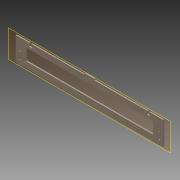
# Autodesk Inventor part: Panel_front
Saved by Autodesk Inventor 2013 (Build 170138000, 138)
## iProperties
Created: 2013-02-02
Part Number: Panel_front
Material: Aluminum 6061
Document SubType Name: Modeling
Designer: xylzlyx
Density: 1 g/cm^3
Author: xylzlyx
Autodesk Inventor part; units mm, degrees
ref_plane "YZ Plane" through (0, 0, 0) normal (1, 0, 0) x (0, 1, 0)
ref_plane "XZ Plane" through (0, 0, 0) normal (0, 1, 0) x (-1, 0, 0)
ref_plane "XY Plane" through (0, 0, 0) normal (0, 0, 1) x (1, 0, 0)
ref_plane "Work Plane1" through (0, 0, -9.525) normal (0, 0, 1) x (1, 0, 0)
sketch "Sketch1" plane through (0, 0, -9.525) normal (0, 0, 1) x (1, 0, 0)
  line L0 (381, -60.8043) -> (381, -64.0283) construction
  line L1 (381, -64.0283) -> (0, -64.0283) construction
  line L2 (0, -64.0283) -> (0, -60.8043) construction
  line L3 (0, -60.8043) -> (381, -60.8043) construction
  line L4 (381, 0) -> (0, 0) construction
  line L5 (0, 0) -> (0, 3.175) construction
  line L6 (0, 3.175) -> (381, 3.175) construction
  line L7 (381, 3.175) -> (381, 0) construction
  line L8 (381, -60.8043) -> (0, -60.8043)
  line L9 (0, -60.8043) -> (0, 0)
  line L10 (0, 0) -> (381, 0)
  line L11 (381, 0) -> (381, -60.8043)
  constraints: 24 end point, 5 horizontal, 4 coincident, 4 vertical, 2 parallel, 1 perpendicular, 8 other
extrude "FrontPanel" add sketch "Sketch1" against normal blind 3.175
fillet "CornerFillet" radius 1 4 edges at (381, -60.8043, -11.1125) (0, -60.8043, -11.1125) (0, 0, -11.1125) (381, 0, -11.1125)
sketch "ScrewSlotSketch" plane through (0, 0, -9.525) normal (0, 0, 1) x (1, 0, 0)
  line L0 (368.3, -28.0035) -> (368.3, -1) projected
  line L1 (12.7, -1) -> (12.7, -28.0035) projected
  line L2 (381, 0) -> (0, 0) construction
  line L3 (0, 0) -> (0, 3.175) construction
  line L4 (0, 3.175) -> (381, 3.175) construction
  line L5 (381, 3.175) -> (381, 0) construction
  line L6 (381, -60.8043) -> (381, -64.0283) construction
  line L7 (381, -64.0283) -> (0, -64.0283) construction
  line L8 (0, -64.0283) -> (0, -60.8043) construction
  line L9 (0, -60.8043) -> (381, -60.8043) construction
  line L10 (344.7987, -8.89) -> (344.7987, 3.175)
  line L11 (344.7987, 3.175) -> (341.0014, 3.175)
  line L12 (341.0014, 3.175) -> (341.0014, -8.89)
  line L13 (341.0014, -8.89) -> (344.7987, -8.89)
  line L14 (346.9958, -8.89) -> (338.8043, -8.89)
  line L15 (338.8043, -8.89) -> (338.8043, -5.8579)
  line L16 (338.8043, -5.8579) -> (346.9958, -5.8579)
  line L17 (346.9958, -5.8579) -> (346.9958, -8.89)
  line L18 (36.2014, -8.89) -> (39.9987, -8.89)
  line L19 (39.9987, -8.89) -> (39.9987, 3.175)
  line L20 (39.9987, 3.175) -> (36.2014, 3.175)
  line L21 (36.2014, 3.175) -> (36.2014, -8.89)
  line L22 (34.0043, -8.89) -> (42.1958, -8.89)
  line L23 (42.1958, -8.89) -> (42.1958, -5.8579)
  line L24 (42.1958, -5.8579) -> (34.0043, -5.8579)
  line L25 (34.0043, -5.8579) -> (34.0043, -8.89)
  point P0 (342.9, 3.175)
  point P1 (342.9, -8.89)
  point P2 (38.1, -8.89)
  point P3 (38.1, 3.175)
  dimension "d4" = 12.065
  dimension "d6" = 3.7973
  dimension "d7" = 25.4
  dimension "d8" = 8.1915
  dimension "d9" = 3.0321
  dimension "d10" = 3.7973
  dimension "d11" = 12.065
  dimension "d12" = 8.1915
  dimension "d13" = 3.0321
  dimension "d14" = 25.4
  constraints: 48 end point, 11 parallel, 6 horizontal, 6 midpoint, 4 vertical, 2 perpendicular, 2 point on line, 1 collinear, 7 other
  measures "d4" distance of L10.start L10.end
  measures "d6" distance of L10.end L11.end
  measures "d7" distance from line of L0 point (342.9, 3.175)
  measures "d8" distance of L14.start L14.end
  measures "d9" distance of L14.end L15.end
  measures "d10" distance of L19.end L20.end
  measures "d11" distance of L20.end L18.start
  measures "d12" distance of L22.start L22.end
  measures "d13" distance of L22.end L23.end
  measures "d14" distance from line of L1 point (38.1, 3.175)
extrude "ScrewSlotExtrusion" cut sketch "ScrewSlotSketch" against normal blind 3.175
fillet "ScrewSlotFillet" radius 0.5 16 edges at (344.7987, 0, -11.1125) (341.0014, 0, -11.1125) (344.7987, -5.8579, -11.1125) (341.0014, -5.8579, -11.1125) (338.8043, -5.8579, -11.1125) (338.8043, -8.89, -11.1125) (346.9958, -8.89, -11.1125) (346.9958, -5.8579, -11.1125) (42.1958, -8.89, -11.1125) (42.1958, -5.8579, -11.1125) (39.9987, -5.8579, -11.1125) (39.9987, 0, -11.1125) (36.2014, 0, -11.1125) (36.2014, -5.8579, -11.1125) (34.0043, -5.8579, -11.1125) (34.0043, -8.89, -11.1125)
sketch "ScrewHoleSketch" plane through (0, 0, -9.525) normal (0, 0, 1) x (1, 0, 0)
  line L0 (34.0043, -8.39) -> (34.0043, -6.3579) projected
  line L1 (368.3, -28.5035) -> (371.475, -28.5035) projected
  line L2 (371.475, -32.3008) -> (368.3, -32.3008) projected
  line L3 (9.525, -28.5035) -> (12.7, -28.5035) projected
  line L4 (12.7, -32.3008) -> (9.525, -32.3008) projected
  line L5 (371.475, -28.5035) -> (371.475, -32.3008) construction
  line L6 (9.525, -28.5035) -> (9.525, -32.3008) construction
  point P0 (0, 0)
  point P1 (11.1125, -30.4021)
  point P2 (369.8875, -30.4021)
  point P3 (369.8875, -28.5035)
  point P4 (371.475, -30.4021)
  point P5 (9.525, -30.4021)
  point P6 (11.1125, -28.5035)
  constraints: 4 end point, 4 midpoint, 2 horizontal alignment, 2 parallel, 2 vertical alignment
hole "ScrewHoles" at (11.1125, -30.4021, -9.525) at (369.8875, -30.4021, -9.525) direction (0, 0, -1) diameter 3.7973 end through all
sketch "BottomTabSketch" plane through (40.4987, 0, -9.525) normal (0, 1, 0) x (1, 0, 0)
  line L0 (162.7014, 3.175) -> (137.3014, 3.175)
  line L1 (137.3014, 3.175) -> (137.3014, 0)
  line L2 (137.3014, 0) -> (162.7014, 0)
  line L3 (162.7014, 0) -> (162.7014, 3.175)
  line L4 (137.0473, 2.929) -> (137.0473, 0.246) projected
  line L5 (137.5473, -0.254) -> (162.4553, -0.254) projected
  point P0 (0, 3.175)
  point P1 (-40.4987, -9.525)
  point P2 (137.3014, 1.5875)
  point P3 (137.0473, 1.5875)
  point P4 (150.0014, 0)
  point P5 (150.0013, -0.254)
  dimension "d29" = 25.4
  constraints: 8 end point, 4 midpoint, 2 horizontal alignment, 2 parallel, 1 horizontal, 1 perpendicular, 1 vertical alignment
  measures "d29" distance of L0.start L0.end
extrude "BottomTab" add sketch "BottomTabSketch" along normal blind 3.175
fillet "BottomTabFillet" radius 0.5 4 edges at (177.8, 0, -11.1125) (177.8, 3.175, -11.1125) (203.2, 3.175, -11.1125) (203.2, 0, -11.1125)
sketch "SlotSketch" plane through (0, 0, -9.525) normal (0, 0, 1) x (1, 0, 0)
  circle A0 centre (11.1125, -30.4021) radius 1.8986 projected
  circle A1 centre (369.8875, -30.4021) radius 1.8986 projected
  line L0 (371.729, -50.6197) -> (368.046, -50.6197)
  line L1 (368.046, -50.6197) -> (368.046, -40.5867)
  line L2 (368.046, -40.5867) -> (371.729, -40.5867)
  line L3 (371.729, -40.5867) -> (371.729, -50.6197)
  line L4 (12.954, -50.6197) -> (9.271, -50.6197)
  line L5 (9.271, -50.6197) -> (9.271, -40.5867)
  line L6 (9.271, -40.5867) -> (12.954, -40.5867)
  line L7 (12.954, -40.5867) -> (12.954, -50.6197)
  line L8 (380, -60.8043) -> (1, -60.8043) projected
  line L9 (203.2, 0.5) -> (203.2, 2.675) projected
  line L10 (11.1125, -30.4021) -> (11.1125, -60.8043) construction
  line L11 (369.8875, -30.4021) -> (369.8875, -60.8043) construction
  point P0 (0, 0)
  point P1 (12.954, -45.6032)
  point P2 (11.1125, -45.6032)
  point P3 (11.1125, -50.6197)
  point P4 (369.8875, -45.6032)
  point P5 (371.729, -45.6032)
  point P6 (369.8875, -50.6197)
  dimension "d34" = 10.033
  dimension "d36" = 3.683
  dimension "d37" = 10.033
  dimension "d38" = 3.683
  constraints: 20 end point, 6 midpoint, 6 parallel, 2 horizontal, 2 horizontal alignment, 2 perpendicular, 2 point on line, 2 vertical alignment
  measures "d34" distance of L0.end L1.end
  measures "d36" distance of L0.start L0.end
  measures "d37" distance of L6.end L4.start
  measures "d38" distance of L4.start L4.end
extrude "Extrusion4" cut sketch "SlotSketch" against normal blind 3.175 contours L0 L1 L2 L3 | L4 L5 L6 L7
fillet "Fillet5" radius 0.5 8 edges at (368.046, -40.5867, -11.1125) (371.729, -40.5867, -11.1125) (371.729, -50.6197, -11.1125) (368.046, -50.6197, -11.1125) (9.271, -40.5867, -11.1125) (12.954, -40.5867, -11.1125) (12.954, -50.6197, -11.1125) (9.271, -50.6197, -11.1125)
sketch "Sketch6" plane through (0, 0, -9.525) normal (0, 0, 1) x (1, 0, 0)
  line L0 (380, -60.8043) -> (1, -60.8043) projected
  line L1 (203.7, 0) -> (340.5014, 0) projected
  circle A0 centre (11.1125, -30.4021) radius 1.8986 projected
  circle A1 centre (369.8875, -30.4021) radius 1.8986 projected
  line L2 (357.1875, -48.1043) -> (23.8125, -48.1043)
  line L3 (23.8125, -48.1043) -> (23.8125, -12.7)
  line L4 (23.8125, -12.7) -> (357.1875, -12.7)
  line L5 (357.1875, -12.7) -> (357.1875, -48.1043)
  point P0 (0, 0)
  dimension "d42" = 12.7
  dimension "d43" = 12.7
  dimension "d44" = 12.7
  dimension "d45" = 12.7
  constraints: 8 end point, 2 parallel, 1 horizontal, 1 perpendicular
  measures "d42" distance from line of L0 L2.start
  measures "d43" distance between parallel lines of L1 L4
  measures "d44" distance from line of A1.centre L5
  measures "d45" distance from line of A0.centre L3
extrude "Extrusion5" cut sketch "Sketch6" against normal blind 25.4 contours L2 L3 L4 L5
fillet "Fillet6" radius 0.5 4 edges at (357.1875, -48.1043, -11.1125) (357.1875, -12.7, -11.1125) (23.8125, -48.1043, -11.1125) (23.8125, -12.7, -11.1125)
equation "\"d4\" = ScrewLen"
equation "\"d6\" = ScrewHoleD"
equation "\"d7\" = ScrewHoleDist"
equation "\"d8\" = NutFlatsGap"
equation "\"d9\" = NutHeightGap"
equation "\"d10\" = ScrewHoleD"
equation "\"d11\" = ScrewLen"
equation "\"d12\" = NutFlatsGap"
equation "\"d13\" = NutHeightGap"
equation "\"d14\" = ScrewHoleDist"
equation "\"d21\" = SlotFilletRad"
equation "\"d22\" = ScrewHoleD"
equation "\"d29\" = TabLength"
equation "\"d33\" = SlotFilletRad"
equation "\"d34\" = SmallSlotLength"
equation "\"d36\" = SlotWidth"
equation "\"d37\" = SmallSlotLength"
equation "\"d38\" = SlotWidth"
equation "\"d41\" = SlotFilletRad"
equation "\"d42\" = EdgeThickness"
equation "\"d43\" = EdgeThickness"
equation "\"d44\" = EdgeThickness"
equation "\"d45\" = EdgeThickness"
equation "\"d48\" = SlotFilletRad"
equation "\"ScrewLen\" = 12.065"
equation "\"ScrewHoleD\" = 3.7973"
equation "\"NutFlatsGap\" = 8.1915"
equation "\"NutHeightGap\" = 3.032125"
equation "\"SlotFilletRad\" = 0.5"
equation "\"TabLength\" = 25.4"
equation "\"SmallSlotLength\" = 10.033"
equation "\"SlotWidth\" = 3.683"
equation "\"EdgeThickness\" = 12.7"
equation "\"ScrewHoleDist\" = 25.4"
body "Solid1"
